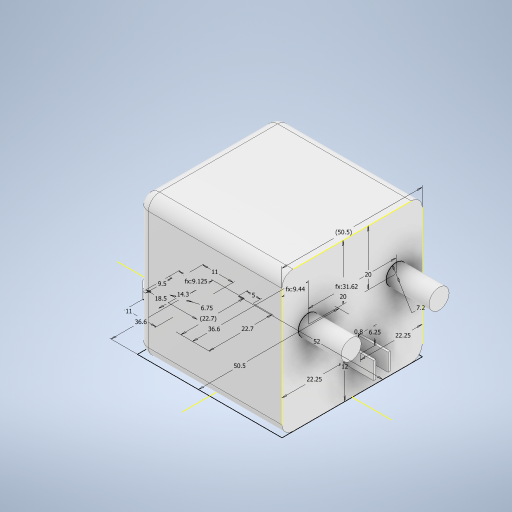
# Autodesk Inventor part: Rapsody-urc
Saved by Autodesk Inventor 2023 (Build 270158000, 158)
## iProperties
Created: 2023-01-10
Part Number: Rapsody-urc
Material: ABS Plastic
Document SubType Name: Modeling
Designer: t205b
Density: 1.06 g/cm^3
Appearance: Smooth - White
Author: t205b
Autodesk Inventor part; units mm, degrees
ref_plane "YZ Plane" through (0, 0, 0) normal (1, 0, 0) x (0, 1, 0)
ref_plane "XZ Plane" through (0, 0, 0) normal (0, 1, 0) x (-1, 0, 0)
ref_plane "XY Plane" through (0, 0, 0) normal (0, 0, 1) x (1, 0, 0)
sketch "Sketch1" plane through (0, 0, 0) normal (0, 1, 0) x (-1, 0, 0)
  line L0 (-26, 25.25) -> (-26, -25.25)
  line L1 (-26, -25.25) -> (26, -25.25)
  line L2 (26, -25.25) -> (26, 25.25)
  line L3 (26, 25.25) -> (-26, 25.25)
  line L4 (26, -11.35) -> (31.1, -7.15)
  line L5 (31.1, -7.15) -> (42.1, -7.15)
  line L6 (42.1, -7.15) -> (44.5, -4.75)
  line L7 (44.5, -4.75) -> (44.5, 4.75)
  line L8 (44.5, 4.75) -> (42.1, 7.15)
  line L9 (42.1, 7.15) -> (31.1, 7.15)
  line L10 (31.1, 7.15) -> (26, 11.35)
  line L11 (0, -35.35) -> (0, 35.35) projected
  line L12 (58.6, 0) -> (-40.1, 0) projected
  circle A0 centre (35.375, 0) radius 3.375
  line L13 (26, -11.35) -> (21, -11.35)
  line L14 (21, -11.35) -> (21, 11.35)
  line L15 (21, 11.35) -> (26, 11.35)
  point P0 (0, 0)
  point P1 (0, -25.25)
  point P2 (36.6, -7.15)
  point P3 (36.6, 7.15)
  point P4 (44.5, 0)
  dimension "d1" = 52
  dimension "d2" = 50.5
  dimension "d3" = 14.3
  dimension "d4" = 36.6
  dimension "d5" = 36.6
  dimension "d6" = 18.5
  dimension "d7" = 9.5
  dimension "d8" = 11
  dimension "d9" = 11
  dimension "d10" = 22.7
  dimension "d11" = 6.75
  dimension "d12" = 9.125
  dimension "d34" = 5
  dimension "d35" = 22.7
  constraints: 28 end point, 7 perpendicular, 4 midpoint, 4 point on line, 2 equal length, 2 parallel, 1 centre point, 1 horizontal, 3 other
  measures "d1" distance between parallel lines of L0 L2
  measures "d2" distance from line of point (0, -25.25) L3
  measures "d3" distance of point (36.6, -7.15) point (36.6, 7.15)
  measures "d4" distance from line of L10.end L1
  measures "d5" distance from line of L3 L4.start
  measures "d6" distance from line of point (44.5, 0) L2
  measures "d7" distance of L6.end L7.end
  measures "d8" distance of L4.end L5.end
  measures "d9" distance of L8.end L9.end
  measures "d10" distance of L10.end L4.start
  measures "d11" diameter of A0
  measures "d12" distance of A0.centre point (44.5, 0)
  measures "d34" distance of L13.start L13.end
  measures "d35" distance of L13.end L14.end
extrude "Extrusion1" add sketch "Sketch1" along normal blind 3.5 contours L14 L15 L2 L12 | L12 L2 L13 L14 | L10 L9 L8 L7 L12 A0 L2 | L12 A0 L7 L6 L5 L4 L2
extrude "Extrusion2" add sketch "Sketch1" along normal blind 50.5 contours L3 L11 L12 L0 | L12 L11 L1 L0 | L3 L2 L15 L14 L12 L11 | L12 L14 L13 L2 L1 L11 | L14 L15 L2 L12 | L12 L2 L13 L14
fillet "Fillet1" radius 4 8 edges at (0, 50.5, 25.25) (-26, 25.25, 25.25) (0, 50.5, -25.25) (-26, 50.5, 0) (0, 0, 25.25) (0, 0, -25.25) (-26, 25.25, -25.25) (-26, 0, -18.3)
sketch "Sketch2" plane through (26, 0, 21.25) normal (1, 0, 0) x (0, 0, -1)
  circle A0 centre (5.44, 30.5) radius 3.6
  circle A1 centre (37.06, 30.5) radius 3.6
  line L0 (18.25, 18.25) -> (19.05, 18.25)
  line L1 (19.05, 18.25) -> (19.05, 12)
  line L2 (19.05, 12) -> (18.25, 12)
  line L3 (18.25, 12) -> (18.25, 18.25)
  line L4 (23.45, 18.25) -> (24.25, 18.25)
  line L5 (24.25, 18.25) -> (24.25, 12)
  line L6 (24.25, 12) -> (23.45, 12)
  line L7 (23.45, 12) -> (23.45, 18.25)
  line L8 (0, 0) -> (42.5, 0) projected
  line L9 (46.5, 4) -> (46.5, 46.5) projected
  line L10 (-4, 4) -> (-4, 46.5) projected
  line L11 (0, 50.5) -> (42.5, 50.5) projected
  point P0 (21.25, 0)
  dimension "d19" = 7.2
  dimension "d20" = 6.25
  dimension "d21" = 0.8
  dimension "d22" = 12
  dimension "d23" = 22.25
  dimension "d24" = 22.25
  dimension "d25" = 31.62
  dimension "d26" = 9.44
  dimension "d27" = 50.5
  dimension "d28" = 20
  dimension "d29" = 20
  constraints: 16 end point, 4 parallel, 2 centre point, 2 horizontal, 2 perpendicular, 2 point on line, 1 collinear, 1 equal radius
  measures "d19" diameter of A1
  measures "d20" distance of L4.end L5.end
  measures "d21" distance of L4.start L4.end
  measures "d22" distance between parallel lines of L2 L8
  measures "d23" distance between parallel lines of L9 L5
  measures "d24" distance between parallel lines of L10 L3
  measures "d25" distance of A1.centre A0.centre
  measures "d26" distance from line of A0.centre L10
  measures "d27" distance between parallel lines of L9 L10
  measures "d28" distance from line of L11 A0.centre
  measures "d29" distance from line of L11 A1.centre
extrude "Extrusion3" add sketch "Sketch2" along normal blind 15.5 contours A0 | A1
extrude "Extrusion4" add sketch "Sketch2" along normal blind 10.75 contours L0 L1 L2 L3 | L4 L5 L6 L7
fillet "Fillet2" radius 4 2 edges at (-24.8284, 1.1716, 24.0784) (-26, 0, 16.3)
equation "\"d26\" = -0.5 * d25 + 0.5 * d27"
body "Solid1"
